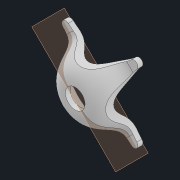
# Autodesk Inventor part: Part1
Saved by Autodesk Inventor 2022 (Build 260153000, 153)
## iProperties
Created: 2021-10-28
Part Number: Part1
Material: 一般
Document SubType Name: Modeling
Designer: Yuta Kage
Density: 1 g/cm^3
Appearance: 既定
Author: Yuta Kage
Autodesk Inventor part; units mm, degrees
ref_plane "XZ Plane" through (0, 0, 0) normal (0, 1, 0) x (-1, 0, 0)
ref_plane "XY Plane" through (0, 0, 0) normal (0, 0, 1) x (1, 0, 0)
sketch "スケッチ1" plane through (0, 0, 0) normal (0, 0, 1) x (1, 0, 0)
  circle A0 centre (0, 0) radius 49 construction
  circle A1 centre (-34.6482, 34.6482) radius 4
  circle A2 centre (-34.6482, -34.6482) radius 4
  circle A3 centre (34.6482, -34.6482) radius 4
  circle A4 centre (34.6482, 34.6482) radius 4
  circle A5 centre (0, 71.8042) radius 46.8042
  circle A6 centre (-71.8042, 0) radius 46.8042
  circle A7 centre (0, -71.8042) radius 46.8042
  circle A8 centre (71.8042, 0) radius 46.8042
  line L0 (-38.6482, -38.6482) -> (38.6482, -38.6482)
  line L1 (38.6482, -38.6482) -> (38.6482, 38.6482)
  line L2 (38.6482, 38.6482) -> (-38.6482, 38.6482)
  line L3 (-38.6482, 38.6482) -> (-38.6482, -38.6482)
  line L4 (-38.6482, -38.6482) -> (38.6482, 38.6482) construction
  line L5 (38.6482, -38.6482) -> (-38.6482, 38.6482) construction
  point P0 (0, 25)
  point P1 (-25, 0)
  point P2 (0, -25)
  point P3 (25, 0)
  point P4 (37.5737, -31.9202)
  point P5 (37.5737, 31.9202)
  point P6 (31.9202, 37.5737)
  point P7 (-31.9202, 37.5737)
  point P8 (-37.5737, 31.9202)
  point P9 (-37.5737, -31.9202)
  point P10 (-31.9202, -37.5737)
  point P11 (31.9202, -37.5737)
  dimension "d0" = 98
  dimension "d1" = 8
  dimension "d4" = 360
  dimension "d6" = 25
  dimension "d9" = 360
  constraints: 12 end point, 4 centre point, 2 midpoint, 2 parallel, 2 tangent, 1 coincident, 1 horizontal, 1 horizontal alignment, 1 perpendicular, 1 vertical alignment, 39 other
  measures "d1" diameter of A1
  measures "d6" distance of point (0, 0) point (0, 25)
extrude "押し出し1" add sketch "スケッチ1" along normal blind 30 contours A1 | A1 A5 A4 A8 A3 A7 A2 A6 | A4 | A2 | A3
ref_plane "作業平面1" through (0, 0, 0) normal (0.7071068, 0.7071068, 0) x (0, 0, 1)
sketch "スケッチ2" plane through (0, 0, 0) normal (0.7071068, 0.7071068, 0) x (0, 0, 1)
  line L0 (0, 53) -> (30, 53) projected
  line L1 (0, 49.1396) -> (0, 53) projected
  line L2 (0, 49.1396) -> (0, 3.9976) projected
  line L3 (30, 49.1396) -> (30, 53) projected
  line L4 (30, 49.1396) -> (30, 3.9976) projected
  line L5 (30, -3.9976) -> (30, 3.9976) projected
  line L6 (0, -3.9976) -> (0, 3.9976) projected
  line L7 (25, 0) -> (25, 10)
  line L8 (25, 10) -> (25, 30.1084) construction
  line L9 (25, 30.1084) -> (0, 24.2541) construction
  line L10 (0, 24.2541) -> (0, 43) construction
  spline S0 degree 3 poles (25, 10) (25, 30.1084) (0, 24.2541) (0, 43) knots 1 1 1 1 2 2 2 2
  line L11 (-8.5053, 0) -> (36.4175, 0) projected
  line L12 (30, 10) -> (30, 0)
  line L13 (5, 43) -> (5, 53)
  spline S1 degree 5 poles (5, 43) (4.9995, 41.9507) (5.0878, 40.9067) (5.2769, 39.8591) (5.9772, 37.9763) (7.233, 36.4173) (7.9139, 35.7734) (9.6317, 34.3839) (11.5277, 33.2409) (12.6405, 32.6191) (15.1414, 31.2724) (17.631, 29.9073) (18.9809, 29.116) (21.8264, 27.2498) (24.3686, 24.9849) (25.6128, 23.6178) (27.9447, 20.3193) (29.3431, 16.5163) (29.7974, 14.3567) (29.9999, 12.1798) (30, 10) knots 0 0 0 0 0 0 0.118738 0.118738 0.118738 0.22413 0.22413 0.22413 0.368663 0.368663 0.368663 0.545774 0.545774 0.545774 0.753163 0.753163 0.753163 1 1 1 1 1 1
  point P0 (0, 0)
  dimension "d14" = 5
  dimension "d15" = 10
  dimension "d16" = 10
  dimension "d17" = 5
  constraints: 6 end point, 3 point on line, 3 vertical, 1 horizontal alignment, 1 midpoint, 1 parallel, 1 perpendicular, 6 other
  measures "d14" distance between parallel lines of L4 L7
  measures "d15" distance from line of L0 L10.end
  measures "d16" distance of L7.start L7.end
  measures "d17" distance between parallel lines of L2 L13
revolve "回転1" cut sketch "スケッチ2" angle 360 about axis through (0, 0, -10) along (0, 0, 1) contours L0 L3 L4 S1 L13 | S0 L7 L11 L6 L2
sketch "スケッチ3" plane through (0, 0, 30) normal (0, 0, 1) x (1, 0, 0)
  circle A0 centre (0, 0) radius 10 projected
  point P0 (7.0711, -7.0711)
  constraints: 1 other
extrude "押し出し2" cut sketch "スケッチ3" against normal blind 30
